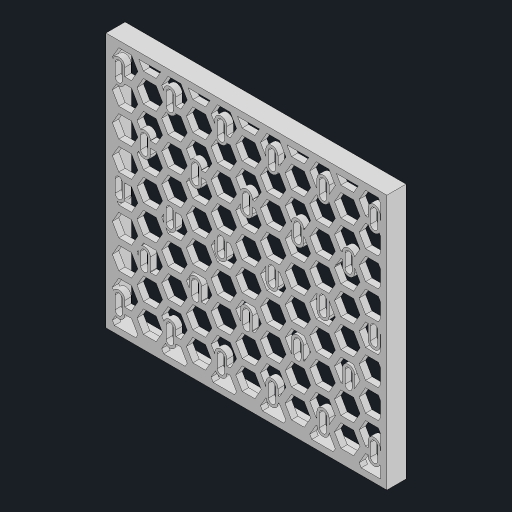
# Autodesk Inventor part: SKÅDIS Pegboard
Saved by Autodesk Inventor 2024 (Build 280153000, 153)
## iProperties
Created: 2024-02-06
Part Number: SKÅDIS Pegboard
Material: 일반
Document SubType Name: Modeling
Designer: KBU
Density: 1 g/cm^3
Appearance: 기본값
Author: KBU
Autodesk Inventor part; units mm, degrees
(part 1 of 3)
ref_plane "YZ Plane" through (0, 0, 0) normal (1, 0, 0) x (0, 1, 0)
ref_plane "XZ Plane" through (0, 0, 0) normal (0, 1, 0) x (-1, 0, 0)
ref_plane "XY Plane" through (0, 0, 0) normal (0, 0, 1) x (1, 0, 0)
sketch "스케치1" plane through (0, 0, 0) normal (0, 0, 1) x (1, 0, 0)
  line L0 (-110, -100) -> (110, -100)
  line L1 (110, -100) -> (110, 100)
  line L2 (110, 100) -> (-110, 100)
  line L3 (-110, 100) -> (-110, -100)
  line L4 (-110, -100) -> (110, 100) construction
  line L5 (110, -100) -> (-110, 100) construction
  line L6 (-100, 74) -> (-100, 84) construction
  line L7 (-102.75, 74) -> (-102.75, 84)
  line L8 (-97.25, 84) -> (-97.25, 74)
  arc A0 (-102.75, 74) -> (-97.25, 74) centre (-100, 74) ccw
  arc A1 (-97.25, 84) -> (-102.75, 84) centre (-100, 84) ccw
  line L9 (-62.75, 74) -> (-62.75, 84)
  line L10 (-60, 74) -> (-60, 84) construction
  line L11 (-57.25, 84) -> (-57.25, 74)
  arc A2 (-62.75, 74) -> (-57.25, 74) centre (-60, 74) ccw
  arc A3 (-57.25, 84) -> (-62.75, 84) centre (-60, 84) ccw
  line L12 (-22.75, 74) -> (-22.75, 84)
  line L13 (-20, 74) -> (-20, 84) construction
  line L14 (-17.25, 84) -> (-17.25, 74)
  arc A4 (-22.75, 74) -> (-17.25, 74) centre (-20, 74) ccw
  arc A5 (-17.25, 84) -> (-22.75, 84) centre (-20, 84) ccw
  line L15 (17.25, 74) -> (17.25, 84)
  line L16 (20, 74) -> (20, 84) construction
  line L17 (22.75, 84) -> (22.75, 74)
  arc A6 (17.25, 74) -> (22.75, 74) centre (20, 74) ccw
  arc A7 (22.75, 84) -> (17.25, 84) centre (20, 84) ccw
  line L18 (57.25, 74) -> (57.25, 84)
  line L19 (60, 74) -> (60, 84) construction
  line L20 (62.75, 84) -> (62.75, 74)
  arc A8 (57.25, 74) -> (62.75, 74) centre (60, 74) ccw
  arc A9 (62.75, 84) -> (57.25, 84) centre (60, 84) ccw
  line L21 (97.25, 74) -> (97.25, 84)
  line L22 (100, 74) -> (100, 84) construction
  line L23 (102.75, 84) -> (102.75, 74)
  arc A10 (97.25, 74) -> (102.75, 74) centre (100, 74) ccw
  arc A11 (102.75, 84) -> (97.25, 84) centre (100, 84) ccw
  line L24 (-80, 34.5) -> (-80, 44.5) construction
  line L25 (-77.25, 34.5) -> (-77.25, 44.5)
  line L26 (-82.75, 44.5) -> (-82.75, 34.5)
  arc A12 (-82.75, 34.5) -> (-77.25, 34.5) centre (-80, 34.5) ccw
  arc A13 (-77.25, 44.5) -> (-82.75, 44.5) centre (-80, 44.5) ccw
  arc A14 (-37.25, 44.5) -> (-42.75, 44.5) centre (-40, 44.5) ccw
  line L27 (-42.75, 44.5) -> (-42.75, 34.5)
  line L28 (-40, 34.5) -> (-40, 44.5) construction
  arc A15 (-42.75, 34.5) -> (-37.25, 34.5) centre (-40, 34.5) ccw
  line L29 (-37.25, 34.5) -> (-37.25, 44.5)
  arc A16 (2.75, 44.5) -> (-2.75, 44.5) centre (0, 44.5) ccw
  line L30 (-2.75, 44.5) -> (-2.75, 34.5)
  line L31 (0, 34.5) -> (0, 44.5) construction
  arc A17 (-2.75, 34.5) -> (2.75, 34.5) centre (0, 34.5) ccw
  line L32 (2.75, 34.5) -> (2.75, 44.5)
  arc A18 (42.75, 44.5) -> (37.25, 44.5) centre (40, 44.5) ccw
  line L33 (37.25, 44.5) -> (37.25, 34.5)
  line L34 (40, 34.5) -> (40, 44.5) construction
  arc A19 (37.25, 34.5) -> (42.75, 34.5) centre (40, 34.5) ccw
  line L35 (42.75, 34.5) -> (42.75, 44.5)
  arc A20 (82.75, 44.5) -> (77.25, 44.5) centre (80, 44.5) ccw
  line L36 (77.25, 44.5) -> (77.25, 34.5)
  line L37 (80, 34.5) -> (80, 44.5) construction
  arc A21 (77.25, 34.5) -> (82.75, 34.5) centre (80, 34.5) ccw
  line L38 (82.75, 34.5) -> (82.75, 44.5)
  line L39 (-100, -5) -> (-100, 5) construction
  line L40 (-102.75, -5) -> (-102.75, 5)
  arc A22 (-102.75, -5) -> (-97.25, -5) centre (-100, -5) ccw
  arc A23 (-97.25, 5) -> (-102.75, 5) centre (-100, 5) ccw
  line L41 (-97.25, 5) -> (-97.25, -5)
  line L42 (-62.75, -5) -> (-62.75, 5)
  line L43 (-60, -5) -> (-60, 5) construction
  arc A24 (-57.25, 5) -> (-62.75, 5) centre (-60, 5) ccw
  line L44 (-57.25, 5) -> (-57.25, -5)
  arc A25 (-62.75, -5) -> (-57.25, -5) centre (-60, -5) ccw
  line L45 (-22.75, -5) -> (-22.75, 5)
  line L46 (-20, -5) -> (-20, 5) construction
  line L47 (-17.25, 5) -> (-17.25, -5)
  arc A26 (-22.75, -5) -> (-17.25, -5) centre (-20, -5) ccw
  arc A27 (-17.25, 5) -> (-22.75, 5) centre (-20, 5) ccw
  line L48 (17.25, -5) -> (17.25, 5)
  line L49 (20, -5) -> (20, 5) construction
  arc A28 (17.25, -5) -> (22.75, -5) centre (20, -5) ccw
  line L50 (22.75, 5) -> (22.75, -5)
  arc A29 (22.75, 5) -> (17.25, 5) centre (20, 5) ccw
  line L51 (57.25, -5) -> (57.25, 5)
  line L52 (60, -5) -> (60, 5) construction
  line L53 (62.75, 5) -> (62.75, -5)
  arc A30 (57.25, -5) -> (62.75, -5) centre (60, -5) ccw
  arc A31 (62.75, 5) -> (57.25, 5) centre (60, 5) ccw
  line L54 (97.25, -5) -> (97.25, 5)
  line L55 (100, -5) -> (100, 5) construction
  arc A32 (97.25, -5) -> (102.75, -5) centre (100, -5) ccw
  line L56 (102.75, 5) -> (102.75, -5)
  arc A33 (102.75, 5) -> (97.25, 5) centre (100, 5) ccw
  line L57 (-100, -84) -> (-100, -74) construction
  line L58 (-102.75, -84) -> (-102.75, -74)
  arc A34 (-102.75, -84) -> (-97.25, -84) centre (-100, -84) ccw
  arc A35 (-97.25, -74) -> (-102.75, -74) centre (-100, -74) ccw
  line L59 (-97.25, -74) -> (-97.25, -84)
  line L60 (-62.75, -84) -> (-62.75, -74)
  line L61 (-60, -84) -> (-60, -74) construction
  arc A36 (-57.25, -74) -> (-62.75, -74) centre (-60, -74) ccw
  line L62 (-57.25, -74) -> (-57.25, -84)
  arc A37 (-62.75, -84) -> (-57.25, -84) centre (-60, -84) ccw
  line L63 (-22.75, -84) -> (-22.75, -74)
  line L64 (-20, -84) -> (-20, -74) construction
  line L65 (-17.25, -74) -> (-17.25, -84)
  arc A38 (-22.75, -84) -> (-17.25, -84) centre (-20, -84) ccw
  arc A39 (-17.25, -74) -> (-22.75, -74) centre (-20, -74) ccw
  line L66 (17.25, -84) -> (17.25, -74)
  line L67 (20, -84) -> (20, -74) construction
  arc A40 (17.25, -84) -> (22.75, -84) centre (20, -84) ccw
  line L68 (22.75, -74) -> (22.75, -84)
  arc A41 (22.75, -74) -> (17.25, -74) centre (20, -74) ccw
  line L69 (57.25, -84) -> (57.25, -74)
  line L70 (60, -84) -> (60, -74) construction
  line L71 (62.75, -74) -> (62.75, -84)
  arc A42 (57.25, -84) -> (62.75, -84) centre (60, -84) ccw
  arc A43 (62.75, -74) -> (57.25, -74) centre (60, -74) ccw
  line L72 (97.25, -84) -> (97.25, -74)
  line L73 (100, -84) -> (100, -74) construction
  arc A44 (97.25, -84) -> (102.75, -84) centre (100, -84) ccw
  line L74 (102.75, -74) -> (102.75, -84)
  arc A45 (102.75, -74) -> (97.25, -74) centre (100, -74) ccw
  line L75 (-80, -44.5) -> (-80, -34.5) construction
  line L76 (-77.25, -44.5) -> (-77.25, -34.5)
  arc A46 (-82.75, -44.5) -> (-77.25, -44.5) centre (-80, -44.5) ccw
  arc A47 (-77.25, -34.5) -> (-82.75, -34.5) centre (-80, -34.5) ccw
  line L77 (-82.75, -34.5) -> (-82.75, -44.5)
  arc A48 (2.75, -34.5) -> (-2.75, -34.5) centre (0, -34.5) ccw
  line L78 (2.75, -44.5) -> (2.75, -34.5)
  line L79 (0, -44.5) -> (0, -34.5) construction
  line L80 (-2.75, -34.5) -> (-2.75, -44.5)
  arc A49 (-2.75, -44.5) -> (2.75, -44.5) centre (0, -44.5) ccw
  arc A50 (42.75, -34.5) -> (37.25, -34.5) centre (40, -34.5) ccw
  line L81 (37.25, -34.5) -> (37.25, -44.5)
  line L82 (40, -44.5) -> (40, -34.5) construction
  line L83 (42.75, -44.5) -> (42.75, -34.5)
  arc A51 (37.25, -44.5) -> (42.75, -44.5) centre (40, -44.5) ccw
  arc A52 (82.75, -34.5) -> (77.25, -34.5) centre (80, -34.5) ccw
  line L84 (80, -44.5) -> (80, -34.5) construction
  line L85 (77.25, -34.5) -> (77.25, -44.5)
  arc A53 (77.25, -44.5) -> (82.75, -44.5) centre (80, -44.5) ccw
  line L86 (82.75, -44.5) -> (82.75, -34.5)
  arc A54 (-37.25, -34.5) -> (-42.75, -34.5) centre (-40, -34.5) ccw
  line L87 (-42.75, -34.5) -> (-42.75, -44.5)
  line L88 (-40, -44.5) -> (-40, -34.5) construction
  arc A55 (-42.75, -44.5) -> (-37.25, -44.5) centre (-40, -44.5) ccw
  line L89 (-37.25, -44.5) -> (-37.25, -34.5)
  line L90 (70, -100) -> (70, 100)
  line L91 (-85, 86.3397) -> (-90, 77.6795)
  line L92 (-90, 77.6795) -> (-100, 77.6795)
  line L93 (-100, 77.6795) -> (-105, 86.3397)
  line L94 (-105, 86.3397) -> (-100, 95)
  line L95 (-100, 95) -> (-90, 95)
  line L96 (-90, 95) -> (-85, 86.3397)
  line L97 (-80.6699, 66.5192) -> (-85.6699, 75.1795)
  line L98 (-85.6699, 75.1795) -> (-80.6699, 83.8397)
  line L99 (-80.6699, 83.8397) -> (-70.6699, 83.8397)
  line L100 (-70.6699, 83.8397) -> (-65.6699, 75.1795)
  line L101 (-65.6699, 75.1795) -> (-70.6699, 66.5192)
  line L102 (-70.6699, 66.5192) -> (-80.6699, 66.5192)
  line L103 (-80.6699, 83.8397) -> (-84.6608, 83.8397) construction
  line L104 (-85, 86.3397) -> (-83.394, 83.5581) construction
  line L105 (-65.6699, 97.5) -> (-70.6699, 88.8397)
  line L106 (-70.6699, 88.8397) -> (-80.6699, 88.8397)
  line L107 (-80.6699, 88.8397) -> (-85.6699, 97.5)
  line L108 (-85.6699, 97.5) -> (-80.6699, 106.1603)
  line L109 (-80.6699, 106.1603) -> (-70.6699, 106.1603)
  line L110 (-70.6699, 106.1603) -> (-65.6699, 97.5)
  line L111 (-164.6517, 120.5465) -> (-169.6517, 111.8863)
  line L112 (-169.6517, 111.8863) -> (-179.6517, 111.8863)
  line L113 (-179.6517, 111.8863) -> (-184.6517, 120.5465)
  line L114 (-184.6517, 120.5465) -> (-179.6517, 129.2068)
  line L115 (-179.6517, 129.2068) -> (-169.6517, 129.2068)
  line L116 (-169.6517, 129.2068) -> (-164.6517, 120.5465)
  line L117 (-119.3301, 88.8397) -> (-124.3301, 97.5)
  line L118 (-109.3301, 88.8397) -> (-119.3301, 88.8397)
  line L119 (-104.3301, 97.5) -> (-109.3301, 88.8397)
  line L120 (-119.3301, 106.1603) -> (-109.3301, 106.1603)
  line L121 (-109.3301, 106.1603) -> (-104.3301, 97.5)
  line L122 (-124.3301, 97.5) -> (-119.3301, 106.1603)
  line L123 (-100, 100) -> (-105, 108.6603)
  line L124 (-90, 100) -> (-100, 100)
  line L125 (-85, 108.6603) -> (-90, 100)
  line L126 (-100, 117.3205) -> (-90, 117.3205)
  line L127 (-90, 117.3205) -> (-85, 108.6603)
  line L128 (-105, 108.6603) -> (-100, 117.3205)
  line L129 (-85, 64.0192) -> (-90, 55.359)
  line L130 (-90, 55.359) -> (-100, 55.359)
  line L131 (-100, 55.359) -> (-105, 64.0192)
  line L132 (-105, 64.0192) -> (-100, 72.6795)
  line L133 (-100, 72.6795) -> (-90, 72.6795)
  line L134 (-90, 72.6795) -> (-85, 64.0192)
  line L135 (-85, 86.3397) -> (-90, 77.6795)
  line L136 (-90, 77.6795) -> (-100, 77.6795)
  line L137 (-100, 77.6795) -> (-105, 86.3397)
  line L138 (-105, 86.3397) -> (-100, 95)
  line L139 (-100, 95) -> (-90, 95)
  line L140 (-90, 95) -> (-85, 86.3397)
  line L141 (-70.6699, 61.5192) -> (-65.6699, 52.859)
  line L142 (-65.6699, 52.859) -> (-70.6699, 44.1987)
  line L143 (-70.6699, 44.1987) -> (-80.6699, 44.1987)
  line L144 (-80.6699, 44.1987) -> (-85.6699, 52.859)
  line L145 (-85.6699, 52.859) -> (-80.6699, 61.5192)
  line L146 (-80.6699, 61.5192) -> (-70.6699, 61.5192)
  line L147 (-90, 72.6795) -> (-85, 64.0192)
  line L148 (-85, 64.0192) -> (-90, 55.359)
  line L149 (-90, 55.359) -> (-100, 55.359)
  line L150 (-100, 55.359) -> (-105, 64.0192)
  line L151 (-105, 64.0192) -> (-100, 72.6795)
  line L152 (-100, 72.6795) -> (-90, 72.6795)
  line L153 (-61.3397, 72.6795) -> (-51.3397, 72.6795)
  line L154 (-51.3397, 72.6795) -> (-46.3397, 64.0192)
  line L155 (-46.3397, 64.0192) -> (-51.3397, 55.359)
  line L156 (-51.3397, 55.359) -> (-61.3397, 55.359)
  line L157 (-61.3397, 55.359) -> (-66.3397, 64.0192)
  line L158 (-66.3397, 64.0192) -> (-61.3397, 72.6795)
  line L159 (-80.6699, 61.5192) -> (-70.6699, 61.5192)
  line L160 (-70.6699, 61.5192) -> (-65.6699, 52.859)
  line L161 (-65.6699, 52.859) -> (-70.6699, 44.1987)
  line L162 (-70.6699, 44.1987) -> (-80.6699, 44.1987)
  line L163 (-80.6699, 44.1987) -> (-85.6699, 52.859)
  line L164 (-85.6699, 52.859) -> (-80.6699, 61.5192)
  line L165 (-66.3397, 86.3397) -> (-61.3397, 95)
  line L166 (-61.3397, 95) -> (-51.3397, 95)
  line L167 (-51.3397, 95) -> (-46.3397, 86.3397)
  line L168 (-46.3397, 86.3397) -> (-51.3397, 77.6795)
  line L169 (-51.3397, 77.6795) -> (-61.3397, 77.6795)
  line L170 (-61.3397, 77.6795) -> (-66.3397, 86.3397)
  line L171 (-66.3397, 64.0192) -> (-61.3397, 72.6795)
  line L172 (-61.3397, 72.6795) -> (-51.3397, 72.6795)
  line L173 (-51.3397, 72.6795) -> (-46.3397, 64.0192)
  line L174 (-46.3397, 64.0192) -> (-51.3397, 55.359)
  line L175 (-51.3397, 55.359) -> (-61.3397, 55.359)
  line L176 (-61.3397, 55.359) -> (-66.3397, 64.0192)
  line L177 (-80.6699, 88.8397) -> (-85.6699, 97.5)
  line L178 (-85.6699, 97.5) -> (-80.6699, 106.1603)
  line L179 (-80.6699, 106.1603) -> (-70.6699, 106.1603)
  line L180 (-70.6699, 106.1603) -> (-65.6699, 97.5)
  line L181 (-65.6699, 97.5) -> (-70.6699, 88.8397)
  line L182 (-70.6699, 88.8397) -> (-80.6699, 88.8397)
  line L183 (-61.3397, 77.6795) -> (-66.3397, 86.3397)
  line L184 (-66.3397, 86.3397) -> (-61.3397, 95)
  line L185 (-61.3397, 95) -> (-51.3397, 95)
  line L186 (-51.3397, 95) -> (-46.3397, 86.3397)
  line L187 (-46.3397, 86.3397) -> (-51.3397, 77.6795)
  line L188 (-51.3397, 77.6795) -> (-61.3397, 77.6795)
  line L189 (-109.3301, 83.8397) -> (-104.3301, 75.1795)
  line L190 (-104.3301, 75.1795) -> (-109.3301, 66.5192)
  line L191 (-109.3301, 66.5192) -> (-119.3301, 66.5192)
  line L192 (-119.3301, 66.5192) -> (-124.3301, 75.1795)
  line L193 (-124.3301, 75.1795) -> (-119.3301, 83.8397)
  line L194 (-119.3301, 83.8397) -> (-109.3301, 83.8397)
  line L195 (-42.0096, 66.5192) -> (-47.0096, 75.1795)
  line L196 (-32.0096, 66.5192) -> (-42.0096, 66.5192)
  line L197 (-27.0096, 75.1795) -> (-32.0096, 66.5192)
  line L198 (-42.0096, 83.8397) -> (-32.0096, 83.8397)
  line L199 (-32.0096, 83.8397) -> (-27.0096, 75.1795)
  line L200 (-47.0096, 75.1795) -> (-42.0096, 83.8397)
  line L201 (-47.0096, 52.859) -> (-42.0096, 61.5192)
  line L202 (-42.0096, 44.1987) -> (-47.0096, 52.859)
  line L203 (-32.0096, 44.1987) -> (-42.0096, 44.1987)
  line L204 (-27.0096, 52.859) -> (-32.0096, 44.1987)
  line L205 (-32.0096, 61.5192) -> (-27.0096, 52.859)
  line L206 (-42.0096, 61.5192) -> (-32.0096, 61.5192)
  line L207 (-22.6795, 55.359) -> (-27.6795, 64.0192)
  line L208 (-12.6795, 55.359) -> (-22.6795, 55.359)
  line L209 (-7.6795, 64.0192) -> (-12.6795, 55.359)
  line L210 (-12.6795, 72.6795) -> (-7.6795, 64.0192)
  line L211 (-22.6795, 72.6795) -> (-12.6795, 72.6795)
  line L212 (-27.6795, 64.0192) -> (-22.6795, 72.6795)
  line L213 (-12.6795, 77.6795) -> (-22.6795, 77.6795)
  line L214 (-7.6795, 86.3397) -> (-12.6795, 77.6795)
  line L215 (-12.6795, 95) -> (-7.6795, 86.3397)
  line L216 (-22.6795, 95) -> (-12.6795, 95)
  line L217 (-27.6795, 86.3397) -> (-22.6795, 95)
  line L218 (-22.6795, 77.6795) -> (-27.6795, 86.3397)
  line L219 (-27.0096, 97.5) -> (-32.0096, 88.8397)
  line L220 (-32.0096, 106.1603) -> (-27.0096, 97.5)
  line L221 (-42.0096, 106.1603) -> (-32.0096, 106.1603)
  line L222 (-47.0096, 97.5) -> (-42.0096, 106.1603)
  line L223 (-42.0096, 88.8397) -> (-47.0096, 97.5)
  line L224 (-32.0096, 88.8397) -> (-42.0096, 88.8397)
  line L225 (15.981, 95) -> (25.981, 95)
  line L226 (15.981, 95) -> (25.981, 95)
  line L227 (10.981, 86.3397) -> (15.981, 95)
  line L228 (10.981, 86.3397) -> (15.981, 95)
  line L229 (25.981, 95) -> (30.981, 86.3397)
  line L230 (25.981, 95) -> (30.981, 86.3397)
  line L231 (54.6413, 77.6795) -> (49.6413, 86.3397)
  line L232 (54.6413, 77.6795) -> (49.6413, 86.3397)
  line L233 (45.3111, 83.8397) -> (50.3111, 75.1795)
  line L234 (49.6413, 86.3397) -> (54.6413, 95)
  line L235 (49.6413, 86.3397) -> (54.6413, 95)
  line L236 (50.3111, 52.859) -> (45.3111, 44.1987)
  line L237 (50.3111, 52.859) -> (45.3111, 44.1987)
  line L238 (35.3111, 44.1987) -> (30.3111, 52.859)
  line L239 (35.3111, 44.1987) -> (30.3111, 52.859)
  line L240 (45.3111, 44.1987) -> (35.3111, 44.1987)
  line L241 (45.3111, 44.1987) -> (35.3111, 44.1987)
  line L242 (35.3111, 83.8397) -> (45.3111, 83.8397)
  line L243 (50.3111, 97.5) -> (45.3111, 88.8397)
  line L244 (45.3111, 88.8397) -> (35.3111, 88.8397)
  line L245 (35.3111, 88.8397) -> (30.3111, 97.5)
  line L246 (30.3111, 97.5) -> (35.3111, 106.1603)
  line L247 (35.3111, 106.1603) -> (45.3111, 106.1603)
  line L248 (45.3111, 106.1603) -> (50.3111, 97.5)
  line L249 (30.3111, 97.5) -> (35.3111, 106.1603)
  line L250 (35.3111, 88.8397) -> (30.3111, 97.5)
  line L251 (35.3111, 106.1603) -> (45.3111, 106.1603)
  line L252 (45.3111, 88.8397) -> (35.3111, 88.8397)
  line L253 (50.3111, 97.5) -> (45.3111, 88.8397)
  line L254 (45.3111, 106.1603) -> (50.3111, 97.5)
  line L255 (30.3111, 52.859) -> (35.3111, 61.5192)
  line L256 (30.3111, 52.859) -> (35.3111, 61.5192)
  line L257 (45.3111, 61.5192) -> (50.3111, 52.859)
  line L258 (45.3111, 61.5192) -> (50.3111, 52.859)
  line L259 (54.6413, 55.359) -> (49.6413, 64.0192)
  line L260 (35.3111, 61.5192) -> (45.3111, 61.5192)
  line L261 (35.3111, 61.5192) -> (45.3111, 61.5192)
  line L262 (45.3111, 66.5192) -> (35.3111, 66.5192)
  line L263 (30.981, 64.0192) -> (25.981, 55.359)
  line L264 (30.981, 86.3397) -> (25.981, 77.6795)
  line L265 (30.981, 86.3397) -> (25.981, 77.6795)
  line L266 (35.3111, 66.5192) -> (30.3111, 75.1795)
  line L267 (30.3111, 75.1795) -> (35.3111, 83.8397)
  line L268 (25.981, 72.6795) -> (30.981, 64.0192)
  line L269 (25.981, 72.6795) -> (30.981, 64.0192)
  line L270 (10.981, 64.0192) -> (15.981, 72.6795)
  line L271 (10.981, 64.0192) -> (15.981, 72.6795)
  line L272 (30.981, 64.0192) -> (25.981, 55.359)
  line L273 (25.981, 55.359) -> (15.981, 55.359)
  line L274 (25.981, 55.359) -> (15.981, 55.359)
  line L275 (15.981, 55.359) -> (10.981, 64.0192)
  line L276 (15.981, 55.359) -> (10.981, 64.0192)
  line L277 (25.981, 100) -> (15.981, 100)
  line L278 (30.981, 108.6603) -> (25.981, 100)
  line L279 (25.981, 117.3205) -> (30.981, 108.6603)
  line L280 (15.981, 117.3205) -> (25.981, 117.3205)
  line L281 (10.981, 108.6603) -> (15.981, 117.3205)
  line L282 (15.981, 100) -> (10.981, 108.6603)
  line L283 (11.6509, 75.1795) -> (6.6509, 66.5192)
  line L284 (6.6509, 83.8397) -> (11.6509, 75.1795)
  line L285 (-3.3491, 83.8397) -> (6.6509, 83.8397)
  line L286 (-8.3491, 75.1795) -> (-3.3491, 83.8397)
  line L287 (6.6509, 66.5192) -> (-3.3491, 66.5192)
  line L288 (-3.3491, 66.5192) -> (-8.3491, 75.1795)
  line L289 (-3.3491, 88.8397) -> (-8.3491, 97.5)
  line L290 (-8.3491, 97.5) -> (-3.3491, 106.1603)
  line L291 (6.6509, 88.8397) -> (-3.3491, 88.8397)
  line L292 (-3.3491, 106.1603) -> (6.6509, 106.1603)
  line L293 (11.6509, 97.5) -> (6.6509, 88.8397)
  line L294 (6.6509, 106.1603) -> (11.6509, 97.5)
  line L295 (25.981, 77.6795) -> (15.981, 77.6795)
  line L296 (15.981, 72.6795) -> (25.981, 72.6795)
  line L297 (25.981, 77.6795) -> (15.981, 77.6795)
  line L298 (15.981, 72.6795) -> (25.981, 72.6795)
  line L299 (15.981, 77.6795) -> (10.981, 86.3397)
  line L300 (15.981, 77.6795) -> (10.981, 86.3397)
  line L301 (50.3111, 75.1795) -> (45.3111, 66.5192)
  line L302 (54.6413, 72.6795) -> (64.6413, 72.6795)
  line L303 (64.6413, 72.6795) -> (69.6413, 64.0192)
  line L304 (54.6413, 55.359) -> (49.6413, 64.0192)
  line L305 (49.6413, 64.0192) -> (54.6413, 72.6795)
  line L306 (49.6413, 64.0192) -> (54.6413, 72.6795)
  line L307 (64.6413, 55.359) -> (54.6413, 55.359)
  line L308 (64.6413, 55.359) -> (54.6413, 55.359)
  line L309 (69.6413, 64.0192) -> (64.6413, 55.359)
  line L310 (69.6413, 64.0192) -> (64.6413, 55.359)
  line L311 (54.6413, 72.6795) -> (64.6413, 72.6795)
  line L312 (64.6413, 72.6795) -> (69.6413, 64.0192)
  line L313 (64.6413, 77.6795) -> (54.6413, 77.6795)
  line L314 (54.6413, 95) -> (64.6413, 95)
  line L315 (54.6413, 95) -> (64.6413, 95)
  line L316 (64.6413, 77.6795) -> (54.6413, 77.6795)
  line L317 (64.6413, 95) -> (69.6413, 86.3397)
  line L318 (64.6413, 95) -> (69.6413, 86.3397)
  line L319 (69.6413, 86.3397) -> (64.6413, 77.6795)
  line L320 (69.6413, 86.3397) -> (64.6413, 77.6795)
  line L321 (73.9714, 88.8397) -> (68.9714, 97.5)
  line L322 (68.9714, 75.1795) -> (73.9714, 83.8397)
  line L323 (68.9714, 97.5) -> (73.9714, 106.1603)
  line L324 (83.9714, 83.8397) -> (88.9714, 75.1795)
  line L325 (73.9714, 83.8397) -> (83.9714, 83.8397)
  line L326 (83.9714, 88.8397) -> (73.9714, 88.8397)
  line L327 (88.9714, 97.5) -> (83.9714, 88.8397)
  line L328 (73.9714, 106.1603) -> (83.9714, 106.1603)
  line L329 (83.9714, 106.1603) -> (88.9714, 97.5)
  line L330 (73.9714, 66.5192) -> (68.9714, 75.1795)
  line L331 (68.9714, 52.859) -> (73.9714, 61.5192)
  line L332 (73.9714, 44.1987) -> (68.9714, 52.859)
  line L333 (88.9714, 75.1795) -> (83.9714, 66.5192)
  line L334 (83.9714, 66.5192) -> (73.9714, 66.5192)
  line L335 (73.9714, 61.5192) -> (83.9714, 61.5192)
  line L336 (83.9714, 61.5192) -> (88.9714, 52.859)
  line L337 (83.9714, 44.1987) -> (73.9714, 44.1987)
  line L338 (88.9714, 52.859) -> (83.9714, 44.1987)
  line L339 (108.3015, 86.3397) -> (103.3015, 77.6795)
  line L340 (93.3015, 95) -> (103.3015, 95)
  line L341 (103.3015, 77.6795) -> (93.3015, 77.6795)
  line L342 (93.3015, 77.6795) -> (88.3015, 86.3397)
  line L343 (88.3015, 86.3397) -> (93.3015, 95)
  line L344 (103.3015, 95) -> (108.3015, 86.3397)
  line L345 (103.3015, 55.359) -> (93.3015, 55.359)
  line L346 (108.3015, 64.0192) -> (103.3015, 55.359)
  line L347 (93.3015, 55.359) -> (88.3015, 64.0192)
  line L348 (103.3015, 72.6795) -> (108.3015, 64.0192)
  line L349 (93.3015, 72.6795) -> (103.3015, 72.6795)
  line L350 (88.3015, 64.0192) -> (93.3015, 72.6795)
  line L351 (112.6314, 66.5192) -> (107.6314, 75.1795)
  line L352 (122.6314, 66.5192) -> (112.6314, 66.5192)
  line L353 (127.6314, 75.1795) -> (122.6314, 66.5192)
  line L354 (112.6314, 83.8397) -> (122.6314, 83.8397)
  line L355 (122.6314, 83.8397) -> (127.6314, 75.1795)
  line L356 (107.6314, 75.1795) -> (112.6314, 83.8397)
  line L357 (88.3014, 41.6989) -> (93.3014, 50.3592)
  line L358 (93.3014, 33.0387) -> (88.3014, 41.6989)
  line L359 (103.3014, 33.0387) -> (93.3014, 33.0387)
  line L360 (108.3014, 41.6989) -> (103.3014, 33.0387)
  line L361 (103.3014, 50.3592) -> (108.3014, 41.6989)
  line L362 (93.3014, 50.3592) -> (103.3014, 50.3592)
  line L363 (131.9614, 33.0387) -> (126.9614, 41.6989)
  line L364 (141.9614, 33.0387) -> (131.9614, 33.0387)
  line L365 (146.9614, 41.6989) -> (141.9614, 33.0387)
  line L366 (141.9614, 50.3592) -> (146.9614, 41.6989)
  line L367 (131.9614, 50.3592) -> (141.9614, 50.3592)
  line L368 (126.9614, 41.6989) -> (131.9614, 50.3592)
  line L369 (161.2914, 66.5192) -> (151.2914, 66.5192)
  line L370 (166.2914, 75.1795) -> (161.2914, 66.5192)
  line L371 (161.2914, 83.8397) -> (166.2914, 75.1795)
  line L372 (151.2914, 83.8397) -> (161.2914, 83.8397)
  line L373 (146.2914, 75.1795) -> (151.2914, 83.8397)
  line L374 (151.2914, 66.5192) -> (146.2914, 75.1795)
  line L375 (146.9614, 108.66) -> (141.9614, 99.9998)
  line L376 (141.9614, 117.3203) -> (146.9614, 108.66)
  line L377 (131.9614, 117.3203) -> (141.9614, 117.3203)
  line L378 (126.9614, 108.66) -> (131.9614, 117.3203)
  line L379 (131.9614, 99.9998) -> (126.9614, 108.66)
  line L380 (141.9614, 99.9998) -> (131.9614, 99.9998)
  line L381 (103.3014, 117.3203) -> (108.3014, 108.66)
  line L382 (93.3014, 117.3203) -> (103.3014, 117.3203)
  line L383 (88.3014, 108.66) -> (93.3014, 117.3203)
  line L384 (93.3014, 99.9998) -> (88.3014, 108.66)
  line L385 (103.3014, 99.9998) -> (93.3014, 99.9998)
  line L386 (108.3014, 108.66) -> (103.3014, 99.9998)
  line L387 (110, 33.038) -> (-110, 33.038)
  line L388 (88.9714, -14.103) -> (83.9714, -22.7633)
  line L389 (83.9714, -22.7633) -> (73.9714, -22.7633)
  line L390 (73.9714, -22.7633) -> (68.9714, -14.103)
  line L391 (68.9714, -14.103) -> (73.9714, -5.4428)
  line L392 (73.9714, -5.4428) -> (83.9714, -5.4428)
  line L393 (69.6413, -2.9428) -> (64.6413, -11.603)
  line L394 (83.9714, -0.4428) -> (73.9714, -0.4428)
  line L395 (64.6413, 5.7175) -> (69.6413, -2.9428)
  line L396 (73.9714, -0.4428) -> (68.9714, 8.2175)
  line L397 (45.3111, -5.4428) -> (50.3111, -14.103)
  line L398 (45.3111, -5.4428) -> (50.3111, -14.103)
  line L399 (54.6413, -11.603) -> (49.6413, -2.9428)
  line L400 (50.3111, 8.2175) -> (45.3111, -0.4428)
  line L401 (49.6413, -2.9428) -> (54.6413, 5.7175)
  line L402 (54.6413, -11.603) -> (49.6413, -2.9428)
  line L403 (49.6413, -2.9428) -> (54.6413, 5.7175)
  line L404 (64.6413, -11.603) -> (54.6413, -11.603)
  line L405 (64.6413, -11.603) -> (54.6413, -11.603)
  line L406 (69.6413, -2.9428) -> (64.6413, -11.603)
  line L407 (64.6413, 5.7175) -> (69.6413, -2.9428)
  line L408 (30.981, -2.9428) -> (25.981, -11.603)
  line L409 (15.981, -11.603) -> (10.981, -2.9428)
  line L410 (30.981, -2.9428) -> (25.981, -11.603)
  line L411 (15.981, -11.603) -> (10.981, -2.9428)
  line L412 (25.981, -11.603) -> (15.981, -11.603)
  line L413 (25.981, -11.603) -> (15.981, -11.603)
  line L414 (30.3111, -14.103) -> (35.3111, -5.4428)
  line L415 (30.3111, -14.103) -> (35.3111, -5.4428)
  line L416 (83.9714, 16.8777) -> (88.9714, 8.2175)
  line L417 (88.9714, 8.2175) -> (83.9714, -0.4428)
  line L418 (83.9714, -5.4428) -> (88.9714, -14.103)
  line L419 (108.3015, 19.3777) -> (103.3015, 10.7175)
  line L420 (103.3015, 5.7175) -> (108.3015, -2.9428)
  line L421 (108.3015, -2.9428) -> (103.3015, -11.603)
  line L422 (93.3015, 10.7175) -> (88.3015, 19.3777)
  line L423 (103.3015, 10.7175) -> (93.3015, 10.7175)
  line L424 (88.3015, -2.9428) -> (93.3015, 5.7175)
  line L425 (103.3015, -11.603) -> (93.3015, -11.603)
  line L426 (93.3015, -11.603) -> (88.3015, -2.9428)
  line L427 (107.6314, 8.2175) -> (112.6314, 16.8777)
  line L428 (112.6314, -0.4428) -> (107.6314, 8.2175)
  line L429 (122.6314, -0.4428) -> (112.6314, -0.4428)
  line L430 (127.6314, 8.2175) -> (122.6314, -0.4428)
  line L431 (112.6314, 16.8777) -> (122.6314, 16.8777)
  line L432 (122.6314, 16.8777) -> (127.6314, 8.2175)
  line L433 (54.6413, 10.7175) -> (49.6413, 19.3777)
  line L434 (54.6413, 10.7175) -> (49.6413, 19.3777)
  line L435 (68.9714, 8.2175) -> (73.9714, 16.8777)
  line L436 (69.6413, 19.3777) -> (64.6413, 10.7175)
  line L437 (69.6413, 19.3777) -> (64.6413, 10.7175)
  line L438 (45.3111, -22.7633) -> (35.3111, -22.7633)
  line L439 (45.3111, -22.7633) -> (35.3111, -22.7633)
  line L440 (35.3111, -22.7633) -> (30.3111, -14.103)
  line L441 (50.3111, -14.103) -> (45.3111, -22.7633)
  line L442 (50.3111, -14.103) -> (45.3111, -22.7633)
  line L443 (35.3111, -5.4428) -> (45.3111, -5.4428)
  line L444 (35.3111, -5.4428) -> (45.3111, -5.4428)
  line L445 (45.3111, -0.4428) -> (35.3111, -0.4428)
  line L446 (35.3111, -0.4428) -> (30.3111, 8.2175)
  line L447 (35.3111, -22.7633) -> (30.3111, -14.103)
  line L448 (10.981, -2.9428) -> (15.981, 5.7175)
  line L449 (10.981, -2.9428) -> (15.981, 5.7175)
  line L450 (25.981, 5.7175) -> (30.981, -2.9428)
  line L451 (25.981, 5.7175) -> (30.981, -2.9428)
  line L452 (15.981, 10.7175) -> (10.981, 19.3777)
  line L453 (15.981, 10.7175) -> (10.981, 19.3777)
  line L454 (103.3014, 33.0378) -> (93.3014, 33.0378)
  line L455 (93.3014, 50.3583) -> (103.3014, 50.3583)
  line L456 (93.3015, 28.038) -> (103.3015, 28.038)
  line L457 (103.3014, 50.3583) -> (108.3014, 41.698)
  line L458 (108.3014, 41.698) -> (103.3014, 33.0378)
  line L459 (103.3015, 28.038) -> (108.3015, 19.3777)
  line L460 (25.981, 28.038) -> (30.981, 19.3777)
  line L461 (25.981, 28.038) -> (30.981, 19.3777)
  line L462 (45.3111, 16.8777) -> (50.3111, 8.2175)
  line L463 (35.3111, 16.8777) -> (45.3111, 16.8777)
  line L464 (45.3111, 21.8777) -> (35.3111, 21.8777)
  line L465 (35.3111, 21.8777) -> (30.3111, 30.538)
  line L466 (45.3111, 21.8777) -> (35.3111, 21.8777)
  line L467 (30.981, 19.3777) -> (25.981, 10.7175)
  line L468 (30.981, 19.3777) -> (25.981, 10.7175)
  line L469 (30.3111, 8.2175) -> (35.3111, 16.8777)
  line L470 (64.6413, 28.038) -> (69.6413, 19.3777)
  line L471 (64.6413, 28.038) -> (69.6413, 19.3777)
  line L472 (68.9714, 30.538) -> (73.9714, 39.1983)
  line L473 (73.9714, 21.8777) -> (68.9714, 30.538)
  line L474 (73.9714, 39.1983) -> (83.9714, 39.1983)
  line L475 (83.9714, 21.8777) -> (73.9714, 21.8777)
  line L476 (73.9714, 16.8777) -> (83.9714, 16.8777)
  line L477 (88.9714, 30.538) -> (83.9714, 21.8777)
  line L478 (88.3015, 19.3777) -> (93.3015, 28.038)
  line L479 (83.9714, 39.1983) -> (88.9714, 30.538)
  line L480 (88.3014, 41.698) -> (93.3014, 50.3583)
  line L481 (93.3014, 33.0378) -> (88.3014, 41.698)
  line L482 (49.6413, 19.3777) -> (54.6413, 28.038)
  line L483 (49.6413, 19.3777) -> (54.6413, 28.038)
  line L484 (50.3111, 30.538) -> (45.3111, 21.8777)
  line L485 (35.3111, 21.8777) -> (30.3111, 30.538)
  line L486 (30.3111, 30.538) -> (35.3111, 39.1983)
  line L487 (35.3111, 39.1983) -> (45.3111, 39.1983)
  line L488 (45.3111, 39.1983) -> (50.3111, 30.538)
  line L489 (30.3111, 30.538) -> (35.3111, 39.1983)
  line L490 (35.3111, 39.1983) -> (45.3111, 39.1983)
  line L491 (54.6413, 28.038) -> (64.6413, 28.038)
  line L492 (45.3111, 39.1983) -> (50.3111, 30.538)
  line L493 (50.3111, 30.538) -> (45.3111, 21.8777)
  line L494 (54.6413, 28.038) -> (64.6413, 28.038)
  line L495 (15.981, 33.038) -> (10.981, 41.6983)
  line L496 (10.981, 41.6983) -> (15.981, 50.3585)
  line L497 (15.981, 28.038) -> (25.981, 28.038)
  line L498 (15.981, 28.038) -> (25.981, 28.038)
  line L499 (25.981, 33.038) -> (15.981, 33.038)
  line L500 (15.981, 50.3585) -> (25.981, 50.3585)
  line L501 (25.981, 50.3585) -> (30.981, 41.6983)
  line L502 (30.981, 41.6983) -> (25.981, 33.038)
  line L503 (-100, -11.603) -> (-105, -2.9428)
  line L504 (-100, -11.603) -> (-105, -2.9428)
  line L505 (-90, -11.603) -> (-100, -11.603)
  line L506 (-90, -11.603) -> (-100, -11.603)
  line L507 (-46.3397, 19.3777) -> (-51.3397, 10.7175)
  line L508 (-46.3397, 19.3777) -> (-51.3397, 10.7175)
  line L509 (-8.3491, 8.2175) -> (-3.3491, 16.8777)
  line L510 (-3.3491, -0.4428) -> (-8.3491, 8.2175)
  line L511 (6.6509, -0.4428) -> (-3.3491, -0.4428)
  line L512 (11.6509, 8.2175) -> (6.6509, -0.4428)
  line L513 (-3.3491, 16.8777) -> (6.6509, 16.8777)
  line L514 (6.6509, 16.8777) -> (11.6509, 8.2175)
  line L515 (-85.6699, -14.103) -> (-80.6699, -5.4428)
  line L516 (-80.6699, -22.7633) -> (-85.6699, -14.103)
  line L517 (-80.6699, -22.7633) -> (-85.6699, -14.103)
  line L518 (-70.6699, -5.4428) -> (-65.6699, -14.103)
  line L519 (-70.6699, -22.7633) -> (-80.6699, -22.7633)
  line L520 (-70.6699, -22.7633) -> (-80.6699, -22.7633)
  line L521 (-65.6699, -14.103) -> (-70.6699, -22.7633)
  line L522 (-65.6699, -14.103) -> (-70.6699, -22.7633)
  line L523 (-85.6699, -14.103) -> (-80.6699, -5.4428)
  line L524 (-32.0096, -22.7633) -> (-42.0096, -22.7633)
  line L525 (-42.0096, -22.7633) -> (-47.0096, -14.103)
  line L526 (-27.0096, -14.103) -> (-32.0096, -22.7633)
  line L527 (-32.0096, -5.4428) -> (-27.0096, -14.103)
  line L528 (-42.0096, -5.4428) -> (-32.0096, -5.4428)
  line L529 (-47.0096, -14.103) -> (-42.0096, -5.4428)
  line L530 (-46.3397, -2.9428) -> (-51.3397, -11.603)
  line L531 (-46.3397, -2.9428) -> (-51.3397, -11.603)
  line L532 (-12.6795, 28.038) -> (-7.6795, 19.3777)
  line L533 (10.981, 19.3777) -> (15.981, 28.038)
  line L534 (10.981, 19.3777) -> (15.981, 28.038)
  line L535 (6.6509, 39.1983) -> (11.6509, 30.538)
  line L536 (11.6509, 30.538) -> (6.6509, 21.8777)
  line L537 (-8.3491, 30.538) -> (-3.3491, 39.1983)
  line L538 (6.6509, 21.8777) -> (-3.3491, 21.8777)
  line L539 (-3.3491, 21.8777) -> (-8.3491, 30.538)
  line L540 (-3.3491, 39.1983) -> (6.6509, 39.1983)
  line L541 (-7.6795, 19.3777) -> (-12.6795, 10.7175)
  line L542 (-12.6795, 5.7175) -> (-7.6795, -2.9428)
  line L543 (-7.6795, -2.9428) -> (-12.6795, -11.603)
  line L544 (-12.6795, -11.603) -> (-22.6795, -11.603)
  line L545 (-22.6795, -11.603) -> (-27.6795, -2.9428)
  line L546 (-51.3397, 5.7175) -> (-46.3397, -2.9428)
  line L547 (-51.3397, 5.7175) -> (-46.3397, -2.9428)
  line L548 (-42.0096, -0.4428) -> (-47.0096, 8.2175)
  line L549 (-32.0096, -0.4428) -> (-42.0096, -0.4428)
  line L550 (-27.0096, 8.2175) -> (-32.0096, -0.4428)
  line L551 (-47.0096, 8.2175) -> (-42.0096, 16.8777)
  line L552 (-42.0096, 16.8777) -> (-32.0096, 16.8777)
  line L553 (-32.0096, 16.8777) -> (-27.0096, 8.2175)
  line L554 (-51.3397, 28.038) -> (-46.3397, 19.3777)
  line L555 (-22.6795, 28.038) -> (-12.6795, 28.038)
  line L556 (-27.6795, 19.3777) -> (-22.6795, 28.038)
  line L557 (-32.0096, 21.8777) -> (-42.0096, 21.8777)
  line L558 (-27.0096, 30.538) -> (-32.0096, 21.8777)
  line L559 (-32.0096, 39.1983) -> (-27.0096, 30.538)
  line L560 (-42.0096, 21.8777) -> (-47.0096, 30.538)
  line L561 (-42.0096, 39.1983) -> (-32.0096, 39.1983)
  line L562 (-47.0096, 30.538) -> (-42.0096, 39.1983)
  line L563 (-70.6699, 16.8777) -> (-65.6699, 8.2175)
  line L564 (-65.6699, 30.538) -> (-70.6699, 21.8777)
  line L565 (-70.6699, 39.1983) -> (-65.6699, 30.538)
  line L566 (-51.3397, 28.038) -> (-46.3397, 19.3777)
  line L567 (-61.3397, 28.038) -> (-51.3397, 28.038)
  line L568 (-66.3397, 19.3777) -> (-61.3397, 28.038)
  line L569 (-66.3397, 19.3777) -> (-61.3397, 28.038)
  line L570 (-65.6699, 30.538) -> (-70.6699, 21.8777)
  line L571 (-70.6699, 39.1983) -> (-65.6699, 30.538)
  line L572 (-61.3397, 28.038) -> (-51.3397, 28.038)
  line L573 (-65.6699, 8.2175) -> (-70.6699, -0.4428)
  line L574 (-80.6699, -5.4428) -> (-70.6699, -5.4428)
  line L575 (-80.6699, -5.4428) -> (-70.6699, -5.4428)
  line L576 (-70.6699, -5.4428) -> (-65.6699, -14.103)
  line L577 (-51.3397, -11.603) -> (-61.3397, -11.603)
  line L578 (-51.3397, -11.603) -> (-61.3397, -11.603)
  line L579 (-61.3397, -11.603) -> (-66.3397, -2.9428)
  line L580 (-61.3397, -11.603) -> (-66.3397, -2.9428)
  line L581 (-90, 28.038) -> (-85, 19.3777)
  line L582 (-90, 28.038) -> (-85, 19.3777)
  line L583 (-85.6699, 30.538) -> (-80.6699, 39.1983)
  line L584 (-80.6699, 21.8777) -> (-85.6699, 30.538)
  line L585 (-80.6699, 21.8777) -> (-85.6699, 30.538)
  line L586 (-85.6699, 30.538) -> (-80.6699, 39.1983)
  line L587 (-80.6699, 16.8777) -> (-70.6699, 16.8777)
  line L588 (-70.6699, 21.8777) -> (-80.6699, 21.8777)
  line L589 (-70.6699, 21.8777) -> (-80.6699, 21.8777)
  line L590 (-80.6699, 39.1983) -> (-70.6699, 39.1983)
  line L591 (-80.6699, 39.1983) -> (-70.6699, 39.1983)
  line L592 (-90, 33.038) -> (-100, 33.038)
  line L593 (-100, 28.038) -> (-90, 28.038)
  line L594 (-100, 28.038) -> (-90, 28.038)
  line L595 (-85, 19.3777) -> (-90, 10.7175)
  line L596 (-85.6699, 8.2175) -> (-80.6699, 16.8777)
  line L597 (-80.6699, 16.8777) -> (-84.6608, 16.8777) construction
  line L598 (-85, 19.3777) -> (-83.394, 16.5961) construction
  line L599 (-85, 19.3777) -> (-90, 10.7175)
  line L600 (-85, 41.6983) -> (-90, 33.038)
  line L601 (-100, 33.038) -> (-105, 41.6983)
  line L602 (-90, 50.3585) -> (-85, 41.6983)
  line L603 (-100, 50.3585) -> (-90, 50.3585)
  line L604 (-105, 41.6983) -> (-100, 50.3585)
  line L605 (-105, 19.3777) -> (-100, 28.038)
  line L606 (-105, 19.3777) -> (-100, 28.038)
  line L607 (-104.3301, 8.2175) -> (-109.3301, -0.4428)
  line L608 (-109.3301, -0.4428) -> (-119.3301, -0.4428)
  line L609 (-109.3301, 16.8777) -> (-104.3301, 8.2175)
  line L610 (-119.3301, 16.8777) -> (-109.3301, 16.8777)
  line L611 (-124.3301, 8.2175) -> (-119.3301, 16.8777)
  line L612 (-119.3301, -0.4428) -> (-124.3301, 8.2175)
  line L613 (-109.3301, 39.1983) -> (-104.3301, 30.538)
  line L614 (-104.3301, 30.538) -> (-109.3301, 21.8777)
  line L615 (-109.3301, 21.8777) -> (-119.3301, 21.8777)
  line L616 (-119.3301, 39.1983) -> (-109.3301, 39.1983)
  line L617 (-119.3301, 21.8777) -> (-124.3301, 30.538)
  line L618 (-124.3301, 30.538) -> (-119.3301, 39.1983)
  line L619 (-70.6699, -0.4428) -> (-80.6699, -0.4428)
  line L620 (-85, -2.9428) -> (-90, -11.603)
  line L621 (-80.6699, -0.4428) -> (-85.6699, 8.2175)
  line L622 (-90, 5.7175) -> (-85, -2.9428)
  line L623 (-90, 5.7175) -> (-85, -2.9428)
  line L624 (-85, -2.9428) -> (-90, -11.603)
  line L625 (93.3015, 5.7175) -> (103.3015, 5.7175)
  line L626 (-110, -166.962) -> (110, 33.038) construction
  line L627 (64.6413, 10.7175) -> (54.6413, 10.7175)
  line L628 (54.6413, 5.7175) -> (64.6413, 5.7175)
  line L629 (25.981, 10.7175) -> (15.981, 10.7175)
  line L630 (15.981, 5.7175) -> (25.981, 5.7175)
  line L631 (-22.6795, 10.7175) -> (-27.6795, 19.3777)
  line L632 (-12.6795, 10.7175) -> (-22.6795, 10.7175)
  line L633 (-27.6795, -2.9428) -> (-22.6795, 5.7175)
  line L634 (-22.6795, 5.7175) -> (-12.6795, 5.7175)
  line L635 (-61.3397, 10.7175) -> (-66.3397, 19.3777)
  line L636 (-51.3397, 10.7175) -> (-61.3397, 10.7175)
  line L637 (-61.3397, 5.7175) -> (-51.3397, 5.7175)
  line L638 (-66.3397, -2.9428) -> (-61.3397, 5.7175)
  line L639 (110, -166.962) -> (-110, 33.038) construction
  line L640 (-100, 10.7175) -> (-105, 19.3777)
  line L641 (-100, 5.7175) -> (-90, 5.7175)
  line L642 (-105, -2.9428) -> (-100, 5.7175)
  line L643 (-90, 10.7175) -> (-100, 10.7175)
  line L644 (-61.3399, 33.0382) -> (-66.3399, 41.6985)
  line L645 (-51.3399, 33.0382) -> (-61.3399, 33.0382)
  line L646 (-46.3399, 41.6985) -> (-51.3399, 33.0382)
  line L647 (-61.3399, 50.3587) -> (-51.3399, 50.3587)
  line L648 (-51.3399, 50.3587) -> (-46.3399, 41.6985)
  line L649 (-66.3399, 41.6985) -> (-61.3399, 50.3587)
  line L650 (-22.6795, 33.0382) -> (-27.6795, 41.6985)
  line L651 (-12.6795, 33.0382) -> (-22.6795, 33.0382)
  line L652 (-7.6795, 41.6985) -> (-12.6795, 33.0382)
  line L653 (-22.6795, 50.3587) -> (-12.6795, 50.3587)
  line L654 (-12.6795, 50.3587) -> (-7.6795, 41.6985)
  line L655 (-27.6795, 41.6985) -> (-22.6795, 50.3587)
  line L656 (-3.3491, 44.1987) -> (-8.3491, 52.859)
  line L657 (6.6509, 44.1987) -> (-3.3491, 44.1987)
  line L658 (11.6509, 52.859) -> (6.6509, 44.1987)
  line L659 (-3.3491, 61.5192) -> (6.6509, 61.5192)
  line L660 (6.6509, 61.5192) -> (11.6509, 52.859)
  line L661 (-8.3491, 52.859) -> (-3.3491, 61.5192)
  line L662 (54.6413, 33.038) -> (49.6413, 41.6983)
  line L663 (64.6413, 33.038) -> (54.6413, 33.038)
  line L664 (69.6413, 41.6983) -> (64.6413, 33.038)
  line L665 (54.6413, 50.3585) -> (64.6413, 50.3585)
  line L666 (64.6413, 50.3585) -> (69.6413, 41.6983)
  line L667 (49.6413, 41.6983) -> (54.6413, 50.3585)
  line L668 (-119.3301, 44.1987) -> (-124.3301, 52.859)
  line L669 (-109.3301, 44.1987) -> (-119.3301, 44.1987)
  line L670 (-104.3301, 52.859) -> (-109.3301, 44.1987)
  line L671 (-119.3301, 61.5192) -> (-109.3301, 61.5192)
  line L672 (-109.3301, 61.5192) -> (-104.3301, 52.859)
  line L673 (-124.3301, 52.859) -> (-119.3301, 61.5192)
  line L674 (-109.3301, -5.4433) -> (-104.3301, -14.1035)
  line L675 (-104.3301, -14.1035) -> (-109.3301, -22.7638)
  line L676 (-109.3301, -22.7638) -> (-119.3301, -22.7638)
  line L677 (-119.3301, -5.4433) -> (-109.3301, -5.4433)
  line L678 (-124.3301, -14.1035) -> (-119.3301, -5.4433)
  line L679 (-119.3301, -22.7638) -> (-124.3301, -14.1035)
  line L680 (-105, -25.2638) -> (-100, -16.6035)
  line L681 (-100, -16.6035) -> (-90, -16.6035)
  line L682 (-90, -16.6035) -> (-85, -25.2638)
  line L683 (-85, -25.2638) -> (-90, -33.924)
  line L684 (-90, -33.924) -> (-100, -33.924)
  line L685 (-100, -33.924) -> (-105, -25.2638)
  line L686 (-80.6699, -22.7638) -> (-85.6699, -14.1035)
  line L687 (-65.6699, -14.1035) -> (-70.6699, -22.7638)
  line L688 (-70.6699, -5.4433) -> (-65.6699, -14.1035)
  line L689 (-80.6699, -5.4433) -> (-70.6699, -5.4433)
  line L690 (-70.6699, -22.7638) -> (-80.6699, -22.7638)
  line L691 (-85.6699, -14.1035) -> (-80.6699, -5.4433)
  line L692 (-66.3397, -25.2638) -> (-61.3397, -16.6035)
  line L693 (-61.3397, -16.6035) -> (-51.3397, -16.6035)
  line L694 (-51.3397, -16.6035) -> (-46.3397, -25.2638)
  line L695 (-51.3397, -16.6035) -> (-46.3397, -25.2638)
  line L696 (-51.3397, -33.924) -> (-61.3397, -33.924)
  line L697 (-51.3397, -33.924) -> (-61.3397, -33.924)
  line L698 (-61.3397, -33.924) -> (-66.3397, -25.2638)
  line L699 (-61.3397, -33.924) -> (-66.3397, -25.2638)
  line L700 (-46.3397, -25.2638) -> (-51.3397, -33.924)
  line L701 (-47.0096, -14.1035) -> (-42.0096, -5.4433)
  line L702 (-32.0096, -5.4433) -> (-27.0096, -14.1035)
  line L703 (-32.0096, -22.7638) -> (-42.0096, -22.7638)
  line L704 (-27.0096, -14.1035) -> (-32.0096, -22.7638)
  line L705 (-42.0096, -22.7638) -> (-47.0096, -14.1035)
  line L706 (-42.0096, -5.4433) -> (-32.0096, -5.4433)
  line L707 (-12.6795, -33.924) -> (-22.6795, -33.924)
  line L708 (-22.6795, -33.924) -> (-27.6795, -25.2638)
  line L709 (-27.6795, -25.2638) -> (-22.6795, -16.6035)
  line L710 (-7.6795, -25.2638) -> (-12.6795, -33.924)
  line L711 (-12.6795, -16.6035) -> (-7.6795, -25.2638)
  line L712 (-22.6795, -16.6035) -> (-12.6795, -16.6035)
  line L713 (25.981, -11.6035) -> (15.981, -11.6035)
  line L714 (15.981, -16.6035) -> (25.981, -16.6035)
  line L715 (6.6509, -22.7638) -> (-3.3491, -22.7638)
  line L716 (-3.3491, -22.7638) -> (-8.3491, -14.1035)
  line L717 (10.981, -25.2638) -> (15.981, -16.6035)
  line L718 (10.981, -25.2638) -> (15.981, -16.6035)
  line L719 (11.6509, -14.1035) -> (6.6509, -22.7638)
  line L720 (25.981, -16.6035) -> (30.981, -25.2638)
  line L721 (25.981, -16.6035) -> (30.981, -25.2638)
  line L722 (-8.3491, -14.1035) -> (-3.3491, -5.4433)
  line L723 (-3.3491, -5.4433) -> (6.6509, -5.4433)
  line L724 (6.6509, -5.4433) -> (11.6509, -14.1035)
  line L725 (54.6413, -33.924) -> (49.6413, -25.2638)
  line L726 (49.6413, -25.2638) -> (54.6413, -16.6035)
  line L727 (64.6413, -33.924) -> (54.6413, -33.924)
  line L728 (64.6413, -33.924) -> (54.6413, -33.924)
  line L729 (49.6413, -25.2638) -> (54.6413, -16.6035)
  line L730 (35.3111, -22.7638) -> (30.3111, -14.1035)
  line L731 (45.3111, -22.7638) -> (35.3111, -22.7638)
  line L732 (64.6413, -16.6035) -> (69.6413, -25.2638)
  line L733 (50.3111, -14.1035) -> (45.3111, -22.7638)
  line L734 (69.6413, -25.2638) -> (64.6413, -33.924)
  line L735 (73.9714, -27.7638) -> (83.9714, -27.7638)
  line L736 (83.9714, -22.7638) -> (73.9714, -22.7638)
  line L737 (73.9714, -22.7638) -> (68.9714, -14.1035)
  line L738 (45.3111, -5.4433) -> (50.3111, -14.1035)
  line L739 (68.9714, -14.1035) -> (73.9714, -5.4433)
  line L740 (93.3015, -33.924) -> (88.3015, -25.2638)
  line L741 (88.3015, -25.2638) -> (93.3015, -16.6035)
  line L742 (103.3015, -33.924) -> (93.3015, -33.924)
  line L743 (103.3015, -16.6035) -> (108.3015, -25.2638)
  line L744 (108.3015, -25.2638) -> (103.3015, -33.924)
  line L745 (54.6413, -16.6035) -> (64.6413, -16.6035)
  line L746 (73.9714, -5.4433) -> (83.9714, -5.4433)
  line L747 (35.3111, -5.4433) -> (45.3111, -5.4433)
  line L748 (30.3111, -14.1035) -> (35.3111, -5.4433)
  line L749 (15.981, -33.924) -> (10.981, -25.2638)
  line L750 (25.981, -33.924) -> (15.981, -33.924)
  line L751 (25.981, -33.924) -> (15.981, -33.924)
  line L752 (15.981, -33.924) -> (10.981, -25.2638)
  line L753 (69.6413, -25.2638) -> (64.6413, -33.924)
  line L754 (64.6413, -16.6035) -> (69.6413, -25.2638)
  line L755 (35.3111, -27.7638) -> (45.3111, -27.7638)
  line L756 (35.3111, -27.7638) -> (45.3111, -27.7638)
  line L757 (54.6413, -33.924) -> (49.6413, -25.2638)
  line L758 (30.981, -25.2638) -> (25.981, -33.924)
  line L759 (30.981, -25.2638) -> (25.981, -33.924)
  line L760 (103.3015, -11.6035) -> (93.3015, -11.6035)
  line L761 (107.6314, -14.1035) -> (112.6314, -5.4433)
  line L762 (112.6314, -5.4433) -> (122.6314, -5.4433)
  line L763 (112.6314, -22.7638) -> (107.6314, -14.1035)
  line L764 (122.6314, -5.4433) -> (127.6314, -14.1035)
  line L765 (122.6314, -22.7638) -> (112.6314, -22.7638)
  line L766 (127.6314, -14.1035) -> (122.6314, -22.7638)
  line L767 (93.3015, -16.6035) -> (103.3015, -16.6035)
  line L768 (88.9714, -14.1035) -> (83.9714, -22.7638)
  line L769 (83.9714, -5.4433) -> (88.9714, -14.1035)
  line L770 (-109.3301, -27.7643) -> (-104.3301, -36.4245)
  line L771 (-104.3301, -36.4245) -> (-109.3301, -45.0848)
  line L772 (-109.3301, -45.0848) -> (-119.3301, -45.0848)
  line L773 (-119.3301, -27.7643) -> (-109.3301, -27.7643)
  line L774 (-124.3301, -36.4245) -> (-119.3301, -27.7643)
  line L775 (-119.3301, -45.0848) -> (-124.3301, -36.4245)
  line L776 (-105, -47.5848) -> (-100, -38.9245)
  line L777 (-100, -38.9245) -> (-90, -38.9245)
  line L778 (-90, -38.9245) -> (-85, -47.5848)
  line L779 (-85, -47.5848) -> (-90, -56.245)
  line L780 (-90, -56.245) -> (-100, -56.245)
  line L781 (-100, -56.245) -> (-105, -47.5848)
  line L782 (-80.6699, -45.0848) -> (-85.6699, -36.4245)
  line L783 (-65.6699, -36.4245) -> (-70.6699, -45.0848)
  line L784 (-70.6699, -27.7643) -> (-65.6699, -36.4245)
  line L785 (-80.6699, -27.7643) -> (-70.6699, -27.7643)
  line L786 (-70.6699, -45.0848) -> (-80.6699, -45.0848)
  line L787 (-85.6699, -36.4245) -> (-80.6699, -27.7643)
  line L788 (-66.3397, -47.5848) -> (-61.3397, -38.9245)
  line L789 (-61.3397, -38.9245) -> (-51.3397, -38.9245)
  line L790 (-51.3397, -38.9245) -> (-46.3397, -47.5848)
  line L791 (-51.3397, -38.9245) -> (-46.3397, -47.5848)
  line L792 (-51.3397, -56.245) -> (-61.3397, -56.245)
  line L793 (-51.3397, -56.245) -> (-61.3397, -56.245)
  line L794 (-61.3397, -56.245) -> (-66.3397, -47.5848)
  line L795 (-61.3397, -56.245) -> (-66.3397, -47.5848)
  line L796 (-46.3397, -47.5848) -> (-51.3397, -56.245)
  line L797 (-47.0096, -36.4245) -> (-42.0096, -27.7643)
  line L798 (-32.0096, -27.7643) -> (-27.0096, -36.4245)
  line L799 (-32.0096, -45.0848) -> (-42.0096, -45.0848)
  line L800 (-27.0096, -36.4245) -> (-32.0096, -45.0848)
  line L801 (-42.0096, -45.0848) -> (-47.0096, -36.4245)
  line L802 (-42.0096, -27.7643) -> (-32.0096, -27.7643)
  line L803 (-12.6795, -56.245) -> (-22.6795, -56.245)
  line L804 (-22.6795, -56.245) -> (-27.6795, -47.5848)
  line L805 (-27.6795, -47.5848) -> (-22.6795, -38.9245)
  line L806 (-7.6795, -47.5848) -> (-12.6795, -56.245)
  line L807 (-12.6795, -38.9245) -> (-7.6795, -47.5848)
  line L808 (-22.6795, -38.9245) -> (-12.6795, -38.9245)
  line L809 (25.981, -33.9245) -> (15.981, -33.9245)
  line L810 (15.981, -38.9245) -> (25.981, -38.9245)
  line L811 (6.6509, -45.0848) -> (-3.3491, -45.0848)
  line L812 (-3.3491, -45.0848) -> (-8.3491, -36.4245)
  line L813 (10.981, -47.5848) -> (15.981, -38.9245)
  line L814 (10.981, -47.5848) -> (15.981, -38.9245)
  line L815 (11.6509, -36.4245) -> (6.6509, -45.0848)
  line L816 (25.981, -38.9245) -> (30.981, -47.5848)
  line L817 (25.981, -38.9245) -> (30.981, -47.5848)
  line L818 (-8.3491, -36.4245) -> (-3.3491, -27.7643)
  line L819 (-3.3491, -27.7643) -> (6.6509, -27.7643)
  line L820 (6.6509, -27.7643) -> (11.6509, -36.4245)
  line L821 (54.6413, -56.245) -> (49.6413, -47.5848)
  line L822 (49.6413, -47.5848) -> (54.6413, -38.9245)
  line L823 (64.6413, -56.245) -> (54.6413, -56.245)
  line L824 (64.6413, -56.245) -> (54.6413, -56.245)
  line L825 (49.6413, -47.5848) -> (54.6413, -38.9245)
  line L826 (35.3111, -45.0848) -> (30.3111, -36.4245)
  line L827 (45.3111, -45.0848) -> (35.3111, -45.0848)
  line L828 (64.6413, -38.9245) -> (69.6413, -47.5848)
  line L829 (50.3111, -36.4245) -> (45.3111, -45.0848)
  line L830 (69.6413, -47.5848) -> (64.6413, -56.245)
  line L831 (73.9714, -50.0848) -> (83.9714, -50.0848)
  line L832 (83.9714, -45.0848) -> (73.9714, -45.0848)
  line L833 (73.9714, -45.0848) -> (68.9714, -36.4245)
  line L834 (45.3111, -27.7643) -> (50.3111, -36.4245)
  line L835 (68.9714, -36.4245) -> (73.9714, -27.7643)
  line L836 (93.3015, -56.245) -> (88.3015, -47.5848)
  line L837 (88.3015, -47.5848) -> (93.3015, -38.9245)
  line L838 (103.3015, -56.245) -> (93.3015, -56.245)
  line L839 (103.3015, -38.9245) -> (108.3015, -47.5848)
  line L840 (108.3015, -47.5848) -> (103.3015, -56.245)
  line L841 (54.6413, -38.9245) -> (64.6413, -38.9245)
  line L842 (73.9714, -27.7643) -> (83.9714, -27.7643)
  line L843 (35.3111, -27.7643) -> (45.3111, -27.7643)
  line L844 (30.3111, -36.4245) -> (35.3111, -27.7643)
  line L845 (15.981, -56.245) -> (10.981, -47.5848)
  line L846 (25.981, -56.245) -> (15.981, -56.245)
  line L847 (25.981, -56.245) -> (15.981, -56.245)
  line L848 (15.981, -56.245) -> (10.981, -47.5848)
  line L849 (69.6413, -47.5848) -> (64.6413, -56.245)
  line L850 (64.6413, -38.9245) -> (69.6413, -47.5848)
  line L851 (35.3111, -50.0848) -> (45.3111, -50.0848)
  line L852 (35.3111, -50.0848) -> (45.3111, -50.0848)
  line L853 (54.6413, -56.245) -> (49.6413, -47.5848)
  line L854 (30.981, -47.5848) -> (25.981, -56.245)
  line L855 (30.981, -47.5848) -> (25.981, -56.245)
  line L856 (103.3015, -33.9245) -> (93.3015, -33.9245)
  line L857 (107.6314, -36.4245) -> (112.6314, -27.7643)
  line L858 (112.6314, -27.7643) -> (122.6314, -27.7643)
  line L859 (112.6314, -45.0848) -> (107.6314, -36.4245)
  line L860 (122.6314, -27.7643) -> (127.6314, -36.4245)
  line L861 (122.6314, -45.0848) -> (112.6314, -45.0848)
  line L862 (127.6314, -36.4245) -> (122.6314, -45.0848)
  line L863 (93.3015, -38.9245) -> (103.3015, -38.9245)
  line L864 (88.9714, -36.4245) -> (83.9714, -45.0848)
  line L865 (83.9714, -27.7643) -> (88.9714, -36.4245)
  line L866 (-109.3301, -50.0853) -> (-104.3301, -58.7455)
  line L867 (-104.3301, -58.7455) -> (-109.3301, -67.4058)
  line L868 (-109.3301, -67.4058) -> (-119.3301, -67.4058)
  line L869 (-119.3301, -50.0853) -> (-109.3301, -50.0853)
  line L870 (-124.3301, -58.7455) -> (-119.3301, -50.0853)
  line L871 (-119.3301, -67.4058) -> (-124.3301, -58.7455)
  line L872 (-105, -69.9058) -> (-100, -61.2455)
  line L873 (-100, -61.2455) -> (-90, -61.2455)
  line L874 (-90, -61.2455) -> (-85, -69.9058)
  line L875 (-85, -69.9058) -> (-90, -78.566)
  line L876 (-90, -78.566) -> (-100, -78.566)
  line L877 (-100, -78.566) -> (-105, -69.9058)
  line L878 (-80.6699, -67.4058) -> (-85.6699, -58.7455)
  line L879 (-65.6699, -58.7455) -> (-70.6699, -67.4058)
  line L880 (-70.6699, -50.0853) -> (-65.6699, -58.7455)
  line L881 (-80.6699, -50.0853) -> (-70.6699, -50.0853)
  line L882 (-70.6699, -67.4058) -> (-80.6699, -67.4058)